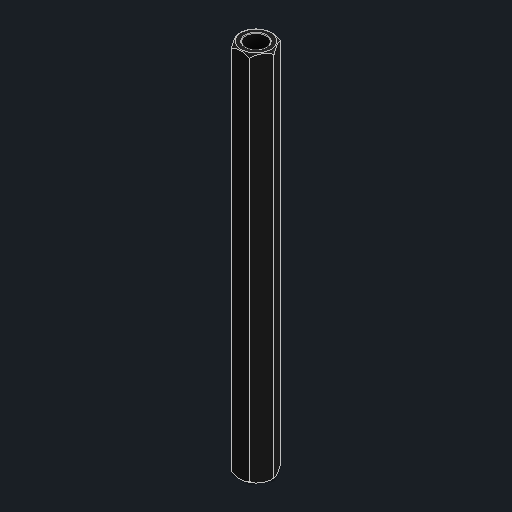
# Autodesk Inventor part: Standoff .5
Saved by Autodesk Inventor 2025.1 (Build 291241000, 241)
## iProperties
Created: 2020-07-20
Part Number: Standoff .5
Material: VEX Aluminum Alloy 5052-H32
Document SubType Name: Modeling
Designer: yuany
Density: 2.68277 g/cm^3
Appearance: Standoffs
Author: yuany
Autodesk Inventor part; units mm, degrees
ref_plane "YZ Plane" through (0, 0, 0) normal (1, 0, 0) x (0, 1, 0)
ref_plane "XZ Plane" through (0, 0, 0) normal (0, 1, 0) x (-1, 0, 0)
ref_plane "XY Plane" through (0, 0, 0) normal (0, 0, 1) x (1, 0, 0)
sketch "Sketch1" plane through (0, 0, 0) normal (0, 1, 0) x (-1, 0, 0)
  line L0 (-1.8331, -3.175) -> (-3.6662, 0)
  line L1 (-3.6662, 0) -> (-1.8331, 3.175)
  line L2 (-1.8331, 3.175) -> (1.8331, 3.175)
  line L3 (1.8331, 3.175) -> (3.6662, 0)
  line L4 (3.6662, 0) -> (1.8331, -3.175)
  line L5 (1.8331, -3.175) -> (-1.8331, -3.175)
  point P0 (0, 0)
  point P1 (0, 0)
  dimension "d0" = 6.35
  constraints: 12 end point, 1 coincident, 1 horizontal, 13 other
  measures "d0" distance between parallel lines of L5 L2
extrude "Body" add sketch "Sketch1" along normal blind 76.2
sketch "Sketch2" plane through (0, 76.2, 0) normal (0, 1, 0) x (1, 0, 0)
  circle A0 centre (0, 0) radius 2.0955
  dimension "d3" = 4.191
  constraints: 1 centre point, 1 coincident
  measures "d3" diameter of A0
extrude "Hole 2" cut sketch "Sketch2" against normal blind 12.7
sketch "Sketch3" plane through (0, 0, 0) normal (0, -1, 0) x (1, 0, 0)
  circle A0 centre (0, 0) radius 2.0955
  dimension "d6" = 4.191
  constraints: 1 centre point, 1 coincident
  measures "d6" diameter of A0
extrude "Hole 1" cut sketch "Sketch3" against normal blind 12.7
chamfer "Hole 2 Chamfer 1" distance 0.127 distance2 0.1244 1 edges at (-2.0955, 76.2, 0) measured on face at (-2.5955, 76.2, 0)
chamfer "Hole 1 Chamfer 1" distance 0.127 distance2 0.1244 1 edges at (-2.0955, 0, 0) measured on face at (-2.5955, 0, 0)
sketch "Sketch4" plane through (0, 0, 0) normal (0, 0, 1) x (1, 0, 0)
  line L0 (1.8331, 76.2) -> (-1.8331, 76.2) projected
  line L1 (0, 76.2) -> (-3.0353, 76.2)
  line L2 (-3.6662, 76.2) -> (-1.8331, 76.2) projected
  line L3 (-3.6662, 0) -> (-3.6662, 76.2) projected
  arc A0 (-3.0353, 76.2) -> (-3.6662, 75.565) centre (-2.2234, 74.7624) ccw
  line L4 (-3.6662, 75.565) -> (-6.3588, 78.1647)
  line L5 (-6.3588, 78.1647) -> (0, 76.2)
  line L6 (0, 76.2) -> (0, 129.864)
  point P0 (0, 0)
  dimension "d15" = 3.0353
  dimension "d16" = 1.651
  dimension "d17" = 0.635
  constraints: 8 end point, 2 point on circle, 2 point on line, 1 centre point, 1 midpoint, 1 vertical
  measures "d15" distance of L1.start L1.end
  measures "d16" radius of A0
  measures "d17" vertical distance of L1.end L4.start
revolve "Hole 2 Chamfer 2" cut sketch "Sketch4" angle 360 about axis through (0, 76.2, 0) along (0, 1, 0)
sketch "Sketch5" plane through (0, 0, 0) normal (0, 0, 1) x (1, 0, 0)
  line L0 (0, 0) -> (-3.0353, 0)
  line L1 (1.8331, 0) -> (-1.8331, 0) projected
  line L2 (-3.6662, 0) -> (-3.6662, 76.2) projected
  arc A0 (-3.6662, 0.635) -> (-3.0353, 0) centre (-2.2234, 1.4376) ccw
  line L3 (0, 0) -> (0, -2.1986)
  line L4 (-3.6662, 0.635) -> (-4.1154, -0.8715)
  line L5 (-4.1154, -0.8715) -> (0, 0)
  point P0 (-3.6662, 75.565)
  dimension "d19" = 3.0353
  dimension "d20" = 1.651
  dimension "d21" = 0.635
  constraints: 8 end point, 2 point on circle, 1 centre point, 1 collinear, 1 point on line, 1 vertical
  measures "d19" distance of L0.start L0.end
  measures "d20" radius of A0
  measures "d21" vertical distance of L0.end L4.start
revolve "Hole 1 Chamfer 2" cut sketch "Sketch5" angle 360 about axis through (0, 0, 0) along (0, -1, 0)
chamfer "Hole 2 Chamfer 1 For Short" [suppressed]
sketch "Sketch7" plane through (0, 0, 0) normal (0, 0, 1) x (1, 0, 0)
  line L0 (0, 76.2004) -> (3.0353, 76.2)
  line L1 (3.6662, 76.2) -> (1.8331, 76.2) projected
  line L2 (3.6662, 0.635) -> (3.6662, 76.2) projected
  arc A0 (3.6662, 75.565) -> (3.0353, 76.2) centre (2.2234, 74.7624) ccw
  line L3 (3.6662, 75.565) -> (4.2663, 77.1032)
  line L4 (4.2663, 77.1032) -> (0, 76.2004)
  line L5 (0, 78.0061) -> (0, 76.2004)
  line L6 (1.8331, 76.2) -> (-1.8331, 76.2) projected
  point P0 (0, 0)
  point P1 (0, 76.2)
  dimension "d33" = 3.0353
  dimension "d34" = 1.651
  dimension "d35" = 0.635
  constraints: 8 end point, 2 point on circle, 2 point on line, 1 centre point, 1 midpoint, 1 perpendicular, 1 vertical alignment
  measures "d33" distance of L0.start L0.end
  measures "d34" radius of A0
  measures "d35" vertical distance of L0.end L3.start
revolve "Hole 2 Chamfer 2 For Short" [suppressed]
body "Solid1"
